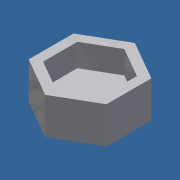
# Autodesk Inventor part: magHexMount
Saved by Autodesk Inventor 2016 (Build 200138000, 138)
## iProperties
Created: 2015-02-14
Part Number: magHexMount
Material: ABS-Kunststoff
Document SubType Name: Modeling
Designer: 4ndreas
Density: 1.06 g/cm^3
Appearance: Glatt - weiß
Mass: 1.27176 g
Surface Area: 12.4397 cm^2
Volume: 1.19977 cm^3
Author: 4ndreas
Autodesk Inventor part; units mm, degrees
ref_plane "YZ Plane" through (0, 0, 0) normal (1, 0, 0) x (0, 1, 0)
ref_plane "XZ Plane" through (0, 0, 0) normal (0, 1, 0) x (-1, 0, 0)
ref_plane "XY Plane" through (0, 0, 0) normal (0, 0, 1) x (1, 0, 0)
sketch "Skizze1" plane through (0, 0, 0) normal (0, 0, 1) x (1, 0, 0)
  circle A0 centre (0, 0) radius 3
  line L0 (0, 9.815) -> (8.5, 4.9075)
  line L1 (8.5, 4.9075) -> (8.5, -4.9075)
  line L2 (8.5, -4.9075) -> (0, -9.815)
  line L3 (0, -9.815) -> (-8.5, -4.9075)
  line L4 (-8.5, -4.9075) -> (-8.5, 4.9075)
  line L5 (-8.5, 4.9075) -> (0, 9.815)
  dimension "d0" = 6
  dimension "d1" = 17
  constraints: 12 end point, 2 coincident, 1 centre point, 1 vertical, 13 other
  measures "d0" diameter of A0
  measures "d1" distance between parallel lines of L1 L4
extrude "Extrusion1" add sketch "Skizze1" along normal blind 2.5
sketch "Skizze2" plane through (0, 0, 2.5) normal (0, 0, 1) x (1, 0, 0)
  line L0 (8.5, 4.9075) -> (0, 9.815) projected
  line L1 (0, 9.815) -> (-8.5, 4.9075) projected
  line L2 (-8.5, 4.9075) -> (-8.5, -4.9075) projected
  line L3 (-8.5, -4.9075) -> (0, -9.815) projected
  line L4 (0, -9.815) -> (8.5, -4.9075) projected
  line L5 (8.5, -4.9075) -> (8.5, 4.9075) projected
extrude "Extrusion2" add sketch "Skizze2" along normal blind 0.5
sketch "Skizze3" plane through (0, 0, 3) normal (0, 0, 1) x (1, 0, 0)
  line L0 (8.5, 4.9075) -> (0, 9.815) projected
  line L1 (0, 9.815) -> (-8.5, 4.9075) projected
  line L2 (-8.5, 4.9075) -> (-8.5, -4.9075) projected
  line L3 (-8.5, -4.9075) -> (0, -9.815) projected
  line L4 (0, -9.815) -> (8.5, -4.9075) projected
  line L5 (8.5, -4.9075) -> (8.5, 4.9075) projected
  line L6 (0, 7.5056) -> (6.5, 3.7528)
  line L7 (6.5, 3.7528) -> (6.5, -3.7528)
  line L8 (6.5, -3.7528) -> (0, -7.5056)
  line L9 (0, -7.5056) -> (-6.5, -3.7528)
  line L10 (-6.5, -3.7528) -> (-6.5, 3.7528)
  line L11 (-6.5, 3.7528) -> (0, 7.5056)
  point P0 (0, 0)
  point P1 (0, 0)
  dimension "d6" = 13
  constraints: 12 end point, 1 coincident, 1 parallel, 13 other
  measures "d6" distance between parallel lines of L7 L10
extrude "Extrusion3" add sketch "Skizze3" along normal blind 5
